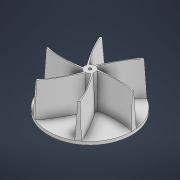
# Autodesk Inventor part: Fan
Saved by Autodesk Inventor 2022 (Build 260153000, 153)
## iProperties
Created: 2022-03-30
Part Number: Fan
Material: 一般
Document SubType Name: Modeling
Designer: neko2
Density: 1 g/cm^3
Appearance: 既定
Author: neko2
Autodesk Inventor part; units mm, degrees
ref_plane "YZ Plane" through (0, 0, 0) normal (1, 0, 0) x (0, 1, 0)
ref_plane "XZ Plane" through (0, 0, 0) normal (0, 1, 0) x (-1, 0, 0)
ref_plane "XY Plane" through (0, 0, 0) normal (0, 0, 1) x (1, 0, 0)
sketch "スケッチ1" plane through (0, 0, 0) normal (0, 1, 0) x (-1, 0, 0)
  circle A0 centre (0, 0) radius 8.75
  dimension "d0" = 17.5
  constraints: 1 centre point, 1 coincident
  measures "d0" diameter of A0
extrude "押し出し1" add sketch "スケッチ1" along normal blind 0.65
sketch "スケッチ3" plane through (0, 0.65, 0) normal (0, 1, 0) x (1, 0, 0)
  line L0 (0.5, 0) -> (5.75, 1) construction
  line L1 (5.75, 1) -> (8.75, 0) construction
  spline S0 degree 2 poles (0.5, 0) (5.75, 1) (8.75, 0) knots 1 1 1 2 2 2
  line L2 (0.5, 1) -> (5.75, 1.5) construction
  line L3 (5.75, 1.5) -> (8.692669, 1) construction
  spline S1 degree 2 poles (0.5, 1) (5.75, 1.5) (8.692669, 1) knots 1 1 1 2 2 2
  line L4 (0.5, 0) -> (0.5, 1)
  line L5 (5.75, 1) -> (5.75, 1.5)
  circle A0 centre (0, 0) radius 8.75
  line L6 (0.25, 0.433013) -> (2.008975, 5.479646) construction
  line L7 (2.008975, 5.479646) -> (4.375, 7.577722) construction
  spline S2 degree 2 poles (0.25, 0.433013) (2.008975, 5.479646) (4.375, 7.577722) knots 1 1 1 2 2 2
  spline S3 degree 2 poles (-0.616025, 0.933013) (1.575962, 5.729646) (3.480309, 8.028072) knots 1 1 1 2 2 2
  line L8 (-0.616025, 0.933013) -> (1.575962, 5.729646) construction
  line L9 (1.575962, 5.729646) -> (3.480309, 8.028072) construction
  line L10 (0.25, 0.433013) -> (-0.616025, 0.933013)
  line L11 (2.008975, 5.479646) -> (1.575962, 5.729646)
  line L12 (-0.25, 0.433013) -> (-3.741025, 4.479646) construction
  line L13 (-3.741025, 4.479646) -> (-4.375, 7.577722) construction
  spline S4 degree 2 poles (-0.25, 0.433013) (-3.741025, 4.479646) (-4.375, 7.577722) knots 1 1 1 2 2 2
  spline S5 degree 2 poles (-1.116025, -0.066987) (-4.174038, 4.229646) (-5.21236, 7.028072) knots 1 1 1 2 2 2
  line L14 (-1.116025, -0.066987) -> (-4.174038, 4.229646) construction
  line L15 (-4.174038, 4.229646) -> (-5.21236, 7.028072) construction
  line L16 (-0.25, 0.433013) -> (-1.116025, -0.066987)
  line L17 (-3.741025, 4.479646) -> (-4.174038, 4.229646)
  line L18 (-0.5, 0) -> (-5.75, -1) construction
  line L19 (-5.75, -1) -> (-8.75, 0) construction
  spline S6 degree 2 poles (-0.5, 0) (-5.75, -1) (-8.75, 0) knots 1 1 1 2 2 2
  spline S7 degree 2 poles (-0.5, -1) (-5.75, -1.5) (-8.692669, -1) knots 1 1 1 2 2 2
  line L20 (-0.5, -1) -> (-5.75, -1.5) construction
  line L21 (-5.75, -1.5) -> (-8.692669, -1) construction
  line L22 (-0.5, 0) -> (-0.5, -1)
  line L23 (-5.75, -1) -> (-5.75, -1.5)
  line L24 (-0.25, -0.433013) -> (-2.008975, -5.479646) construction
  line L25 (-2.008975, -5.479646) -> (-4.375, -7.577722) construction
  spline S8 degree 2 poles (-0.25, -0.433013) (-2.008975, -5.479646) (-4.375, -7.577722) knots 1 1 1 2 2 2
  spline S9 degree 2 poles (0.616025, -0.933013) (-1.575962, -5.729646) (-3.480309, -8.028072) knots 1 1 1 2 2 2
  line L26 (0.616025, -0.933013) -> (-1.575962, -5.729646) construction
  line L27 (-1.575962, -5.729646) -> (-3.480309, -8.028072) construction
  line L28 (-0.25, -0.433013) -> (0.616025, -0.933013)
  line L29 (-2.008975, -5.479646) -> (-1.575962, -5.729646)
  line L30 (0.25, -0.433013) -> (3.741025, -4.479646) construction
  line L31 (3.741025, -4.479646) -> (4.375, -7.577722) construction
  spline S10 degree 2 poles (0.25, -0.433013) (3.741025, -4.479646) (4.375, -7.577722) knots 1 1 1 2 2 2
  spline S11 degree 2 poles (1.116025, 0.066987) (4.174038, -4.229646) (5.21236, -7.028072) knots 1 1 1 2 2 2
  line L32 (1.116025, 0.066987) -> (4.174038, -4.229646) construction
  line L33 (4.174038, -4.229646) -> (5.21236, -7.028072) construction
  line L34 (0.25, -0.433013) -> (1.116025, 0.066987)
  line L35 (3.741025, -4.479646) -> (4.174038, -4.229646)
  point P0 (4.375, 7.577722)
  point P1 (3.480309, 8.028072)
  point P2 (-4.375, 7.577722)
  point P3 (-5.21236, 7.028072)
  point P4 (-8.75, 0)
  point P5 (-8.692669, -1)
  point P6 (-4.375, -7.577722)
  point P7 (-3.480309, -8.028072)
  point P8 (5.21236, -7.028072)
  dimension "d4" = 1
  dimension "d5" = 0.5
  dimension "d6" = 1
  dimension "d8" = 0.5
  dimension "d10" = 1
  dimension "d11" = 3
  dimension "d14" = 360
  constraints: 24 end point, 12 coincident, 2 horizontal alignment, 2 point on circle, 2 vertical, 133 other
  measures "d4" vertical distance of L0.end L0.start
  measures "d5" vertical distance of L2.end L2.start
  measures "d6" distance of L0.start L2.start
  measures "d8" distance from line of L4 point (0, 0)
  measures "d10" vertical distance of L3.end L1.end
  measures "d11" horizontal distance of L1.end L0.end
extrude "押し出し2" add sketch "スケッチ3" along normal blind 7 draft -2.5 contours L4 S1 A0 S0 | A0 S10 L34 S11 | S2 L10 S3 A0 | A0 S8 L28 S9 | S4 L16 S5 A0 | A0 S6 L22 S7
sketch "スケッチ4" plane through (0, 0.65, 0) normal (0, 1, 0) x (1, 0, 0)
  circle A0 centre (0, 0) radius 1.5
  dimension "d18" = 3
  constraints: 1 centre point, 1 coincident
  measures "d18" diameter of A0
extrude "押し出し3" add sketch "スケッチ4" along normal blind 7 draft -3
sketch "スケッチ5" plane through (0, 7.65, 0) normal (0, 1, 0) x (1, 0, 0)
  arc A0 (-0.376264, 1.452042) -> (-0.895615, 1.203276) centre (0, 0) ccw
  circle A1 centre (0, 0) radius 0.3
  dimension "d21" = 0.6
  constraints: 1 centre point, 1 coincident
  measures "d21" diameter of A1
extrude "押し出し4" cut sketch "スケッチ5" against normal through all
